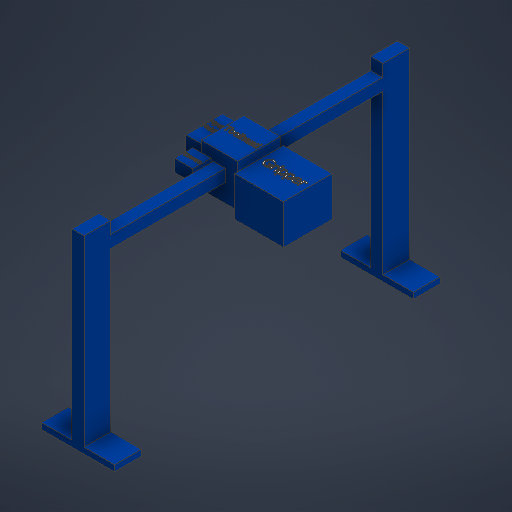
# Autodesk Inventor part: ToolheadMock
Saved by Autodesk Inventor 2025.1 (Build 291241000, 241)
## iProperties
Created: 2024-11-01
Part Number: ToolheadMock
Material: Generic
Document SubType Name: Modeling
Designer: jerem
Density: 1 g/cm^3
Appearance: Default
Author: jerem
Autodesk Inventor part; units mm, degrees
(part 1 of 2)
ref_plane "YZ Plane" through (0, 0, 0) normal (1, 0, 0) x (0, 1, 0)
ref_plane "XZ Plane" through (0, 0, 0) normal (0, 1, 0) x (-1, 0, 0)
sketch "Sketch1" plane through (0, 0, 0) normal (0, 1, 0) x (-1, 0, 0)
  line L0 (0, 0) -> (120, 0)
  line L1 (120, 0) -> (120, -44)
  line L2 (120, -44) -> (0, -44)
  line L3 (0, -44) -> (0, 0)
  line L4 (70, 0) -> (50, 0)
  line L5 (50, 0) -> (50, -44)
  line L6 (50, -44) -> (70, -44)
  line L7 (70, -44) -> (70, 0)
  point P0 (60, -44)
  dimension "d0" = 44
  dimension "d1" = 120
  dimension "d4" = 20
  dimension "d5" = 10
  constraints: 16 end point, 4 parallel, 2 horizontal, 2 perpendicular, 2 point on line, 1 midpoint
  measures "d0" distance of L0.end L1.end
  measures "d1" distance of L0.start L0.end
  measures "d4" distance between parallel lines of L5 L7
  measures "d5" distance from line of L5 point (60, -44)
extrude "Extrusion1" add sketch "Sketch1" along normal blind 10
extrude "Extrusion2" add sketch "Sketch1" along normal blind 300 from surface at 10 contours L0 L7 L2 L5
sketch "Sketch2" plane through (0, 0, -44) normal (0, 0, -1) x (-1, 0, 0)
  line L0 (50, 10) -> (50, 310) projected
  line L1 (70, 310) -> (70, 10) projected
  line L2 (50, 290) -> (70, 290)
  line L3 (70, 290) -> (70, 270)
  line L4 (70, 270) -> (50, 270)
  line L5 (50, 270) -> (50, 290)
  line L6 (70, 310) -> (50, 310) projected
  point P0 (0, 0)
  dimension "d8" = 20
  dimension "d9" = 20
  constraints: 8 end point, 2 parallel, 2 point on line, 1 horizontal, 1 perpendicular
  measures "d8" distance between parallel lines of L4 L2
  measures "d9" distance between parallel lines of L6 L2
extrude "Extrusion3" add sketch "Sketch2" along normal blind 445.8 contours L0 L2 L1 L4
ref_plane "Work Plane1" through (-50, 310, -266.9) normal (0, 0, -1) x (-1, 0, 0)
mirror "Mirror1" about plane through (-50, 310, -266.9) normal (0, 0, -1) of "Extrusion1", "Extrusion2"
sketch "Sketch3" plane through (-50, 310, -266.9) normal (0, 0, -1) x (-1, 0, 0)
  line L0 (40, 0) -> (-20, 0)
  line L1 (-20, 0) -> (-20, -70)
  line L2 (-20, -70) -> (40, -70)
  line L3 (40, -70) -> (40, 0)
  line L4 (20, 0) -> (20, -300) projected
  line L5 (0, -300) -> (0, 0) projected
  line L6 (20, -20) -> (0, -20) projected
  line L7 (0, -40) -> (20, -40) projected
  line L8 (40, -10) -> (70, -10)
  line L9 (70, -10) -> (70, -75)
  line L10 (70, -75) -> (40, -75)
  line L11 (40, -75) -> (40, -10)
  line L12 (-20, -15) -> (-100, -15)
  line L13 (-100, -15) -> (-100, -80)
  line L14 (-100, -80) -> (-20, -80)
  line L15 (-20, -80) -> (-20, -15)
  line L16 (23.5907, -17.4623) -> (53.5907, -17.4623)
  line L17 (53.5907, -17.4623) -> (53.5907, -37.4623)
  line L18 (53.5907, -37.4623) -> (23.5907, -37.4623)
  line L19 (23.5907, -37.4623) -> (23.5907, -17.4623)
  point P0 (-50, -310)
  point P1 (10, -20)
  point P2 (10, 0)
  point P3 (40, -70)
  point P4 (-20, -70)
  dimension "d12" = 20
  dimension "d13" = 20
  dimension "d14" = 20
  dimension "d15" = 30
  dimension "d16" = 10
  dimension "d17" = 15
  dimension "d18" = 10
  dimension "d19" = 80
  dimension "d20" = 30
  dimension "d41" = 5
  dimension "d42" = 30
  dimension "d43" = 20
  constraints: 32 end point, 8 parallel, 4 horizontal, 4 perpendicular, 2 midpoint, 2 point on line
  measures "d12" distance between parallel lines of L4 L3
  measures "d13" distance between parallel lines of L1 L5
  measures "d14" distance of point (10, -20) point (10, 0)
  measures "d15" distance between parallel lines of L2 L7
  measures "d16" distance from line of L0.start L8
  measures "d17" distance between parallel lines of L12 L0
  measures "d18" distance between parallel lines of L2 L14
  measures "d19" distance between parallel lines of L1 L13
  measures "d20" distance between parallel lines of L3 L9
  measures "d41" distance between parallel lines of L2 L10
  measures "d42" distance of L17.end L18.end
  measures "d43" distance of L16.end L17.end
extrude "Extrusion4" add sketch "Sketch3" along normal mid plane 70 contours L3 L16 L19 L18 L2 L4 L0 | L4 L6 L5 L0 | L5 L2 L1 L0 | L3 L18 L19 L16 | L4 L2 L5 L7
extrude "Extrusion5" add sketch "Sketch3" along normal mid plane 60 contours L8 L9 L10 L11 L3 L18 L17 L16 | L16 L17 L18 L3
extrude "Extrusion6" add sketch "Sketch3" along normal mid plane 80 contours L1 L15 L14 L13 L12
sketch "Sketch4" plane through (-30, 295, -306.9) normal (0, 1, 0) x (1, 0, 0)
  line L0 (6.4231, -29.5897) -> (62.2497, -29.5897) construction
  line L1 (62.2497, -29.5897) -> (62.2497, -34.515) construction
  line L2 (62.2497, -34.515) -> (6.4231, -34.515) construction
  line L3 (6.4231, -34.515) -> (6.4231, -29.5897) construction
  spline S0 degree 2 poles (14.227, -45.1488) (12.6346, -45.1488) (9.9969, -44.1764) (9.0487, -43.1918) knots 0 0 0 1 2 2 2
  spline S1 degree 2 poles (9.0487, -43.1918) (8.1006, -42.195) (7.0917, -39.2534) (7.0917, -37.345) knots 0 0 0 1 2 2 2
  spline S2 degree 2 poles (7.0917, -37.345) (7.0917, -35.5338) (8.1128, -32.6651) (9.0609, -31.644) knots 0 0 0 1 2 2 2
  spline S3 degree 2 poles (9.0609, -31.644) (9.9726, -30.6594) (12.6468, -29.5897) (14.2392, -29.5897) knots 0 0 0 1 2 2 2
  spline S4 degree 2 poles (14.2392, -29.5897) (15.005, -29.5897) (16.3907, -29.8085) (17.0228, -30.003) knots 0 0 0 1 2 2 2
  spline S5 degree 2 poles (17.0228, -30.003) (17.5333, -30.1488) (18.7732, -30.6837) (19.15, -30.8782) knots 0 0 0 1 2 2 2
  line L4 (19.15, -30.8782) -> (19.15, -33.285)
  line L5 (19.15, -33.285) -> (18.9799, -33.285)
  spline S6 degree 2 poles (18.9799, -33.285) (18.603, -32.9568) (17.8129, -32.3612) (17.0836, -32.0208) knots 0 0 0 1 2 2 2
  spline S7 degree 2 poles (17.0836, -32.0208) (16.4758, -31.7169) (14.9077, -31.3158) (14.0082, -31.3158) knots 0 0 0 1 2 2 2
  spline S8 degree 2 poles (14.0082, -31.3158) (11.8445, -31.3158) (9.1703, -34.5735) (9.1703, -37.2842) knots 0 0 0 1 2 2 2
  spline S9 degree 2 poles (9.1703, -37.2842) (9.1703, -38.7915) (9.8753, -41.0524) (10.5439, -41.8304) knots 0 0 0 1 2 2 2
  spline S10 degree 2 poles (10.5439, -41.8304) (11.1881, -42.6083) (13.0115, -43.4228) (14.1541, -43.4228) knots 0 0 0 1 2 2 2
  spline S11 degree 2 poles (14.1541, -43.4228) (14.9928, -43.4228) (16.6703, -43.1796) (17.2416, -42.9365) knots 0 0 0 1 2 2 2
  line L6 (17.2416, -42.9365) -> (17.2416, -39.0589)
  line L7 (17.2416, -39.0589) -> (13.7651, -39.0589)
  line L8 (13.7651, -39.0589) -> (13.7651, -37.3085)
  line L9 (13.7651, -37.3085) -> (19.2108, -37.3085)
  line L10 (19.2108, -37.3085) -> (19.2108, -43.8604)
  spline S12 degree 2 poles (19.2108, -43.8604) (18.834, -44.0305) (17.5455, -44.5532) (16.9985, -44.7112) knots 0 0 0 1 2 2 2
  spline S13 degree 2 poles (16.9985, -44.7112) (16.257, -44.93) (15.0658, -45.1488) (14.227, -45.1488) knots 0 0 0 1 2 2 2
  line L11 (27.5374, -35.631) -> (27.4402, -35.631)
  spline S14 degree 2 poles (27.4402, -35.631) (27.2214, -35.5702) (26.7473, -35.5459) (26.4191, -35.5459) knots 0 0 0 1 2 2 2
  spline S15 degree 2 poles (26.4191, -35.5459) (25.6533, -35.5459) (24.146, -36.2145) (23.4653, -36.8709) knots 0 0 0 1 2 2 2
  line L12 (23.4653, -36.8709) -> (23.4653, -44.8571)
  line L13 (23.4653, -44.8571) -> (21.569, -44.8571)
  line L14 (21.569, -44.8571) -> (21.569, -33.601)
  line L15 (21.569, -33.601) -> (23.4653, -33.601)
  line L16 (23.4653, -33.601) -> (23.4653, -35.2785)
  spline S16 degree 2 poles (23.4653, -35.2785) (24.4985, -34.3547) (26.0423, -33.601) (26.7716, -33.601) knots 0 0 0 1 2 2 2
  spline S17 degree 2 poles (26.7716, -33.601) (27.0633, -33.601) (27.3551, -33.6253) (27.5374, -33.6618) knots 0 0 0 1 2 2 2
  line L17 (27.5374, -33.6618) -> (27.5374, -35.631)
  line L18 (30.941, -44.8571) -> (29.0447, -44.8571)
  line L19 (29.0447, -44.8571) -> (29.0447, -33.601)
  line L20 (29.0447, -33.601) -> (30.941, -33.601)
  line L21 (30.941, -33.601) -> (30.941, -44.8571)
  line L22 (31.0747, -31.7291) -> (28.9231, -31.7291)
  line L23 (28.9231, -31.7291) -> (28.9231, -29.7599)
  line L24 (28.9231, -29.7599) -> (31.0747, -29.7599)
  line L25 (31.0747, -29.7599) -> (31.0747, -31.7291)
  spline S18 degree 2 poles (43.1573, -38.9252) (43.1573, -41.7453) (40.471, -45.0759) (38.4167, -45.0759) knots 0 0 0 1 2 2 2
  spline S19 degree 2 poles (38.4167, -45.0759) (37.5779, -45.0759) (36.2894, -44.6869) (35.6209, -44.2858) knots 0 0 0 1 2 2 2
  line L26 (35.6209, -44.2858) -> (35.6209, -49.0022)
  line L27 (35.6209, -49.0022) -> (33.7246, -49.0022)
  line L28 (33.7246, -49.0022) -> (33.7246, -33.601)
  line L29 (33.7246, -33.601) -> (35.6209, -33.601)
  line L30 (35.6209, -33.601) -> (35.6209, -34.7801)
  spline S20 degree 2 poles (35.6209, -34.7801) (36.3259, -34.1359) (38.052, -33.285) (39.0609, -33.285) knots 0 0 0 1 2 2 2
  spline S21 degree 2 poles (39.0609, -33.285) (40.9936, -33.285) (43.1573, -36.3482) (43.1573, -38.9252) knots 0 0 0 1 2 2 2
  spline S22 degree 2 poles (41.2003, -39.144) (41.2003, -37.2112) (39.9726, -35.084) (38.599, -35.084) knots 0 0 0 1 2 2 2
  spline S23 degree 2 poles (38.599, -35.084) (37.7967, -35.084) (36.2894, -35.8012) (35.6209, -36.3604) knots 0 0 0 1 2 2 2
  line L31 (35.6209, -36.3604) -> (35.6209, -42.7542)
  spline S24 degree 2 poles (35.6209, -42.7542) (36.3624, -43.1067) (37.4199, -43.3741) (38.1006, -43.3741) knots 0 0 0 1 2 2 2
  spline S25 degree 2 poles (38.1006, -43.3741) (39.5714, -43.3741) (41.2003, -41.2104) (41.2003, -39.144) knots 0 0 0 1 2 2 2
  spline S26 degree 2 poles (54.5593, -38.9252) (54.5593, -41.7453) (51.8729, -45.0759) (49.8186, -45.0759) knots 0 0 0 1 2 2 2
  spline S27 degree 2 poles (49.8186, -45.0759) (48.9799, -45.0759) (47.6914, -44.6869) (47.0228, -44.2858) knots 0 0 0 1 2 2 2
  line L32 (47.0228, -44.2858) -> (47.0228, -49.0022)
  line L33 (47.0228, -49.0022) -> (45.1265, -49.0022)
  line L34 (45.1265, -49.0022) -> (45.1265, -33.601)
  line L35 (45.1265, -33.601) -> (47.0228, -33.601)
  line L36 (47.0228, -33.601) -> (47.0228, -34.7801)
  spline S28 degree 2 poles (47.0228, -34.7801) (47.7278, -34.1359) (49.4539, -33.285) (50.4628, -33.285) knots 0 0 0 1 2 2 2
  spline S29 degree 2 poles (50.4628, -33.285) (52.3956, -33.285) (54.5593, -36.3482) (54.5593, -38.9252) knots 0 0 0 1 2 2 2
  spline S30 degree 2 poles (52.6022, -39.144) (52.6022, -37.2112) (51.3745, -35.084) (50.0009, -35.084) knots 0 0 0 1 2 2 2
  spline S31 degree 2 poles (50.0009, -35.084) (49.1987, -35.084) (47.6914, -35.8012) (47.0228, -36.3604) knots 0 0 0 1 2 2 2
  line L37 (47.0228, -36.3604) -> (47.0228, -42.7542)
  spline S32 degree 2 poles (47.0228, -42.7542) (47.7643, -43.1067) (48.8218, -43.3741) (49.5026, -43.3741) knots 0 0 0 1 2 2 2
  spline S33 degree 2 poles (49.5026, -43.3741) (50.9734, -43.3741) (52.6022, -41.2104) (52.6022, -39.144) knots 0 0 0 1 2 2 2
  spline S34 degree 2 poles (61.415, -45.1124) (58.7165, -45.1124) (55.7505, -42.0856) (55.7505, -39.2898) knots 0 0 0 1 2 2 2
  spline S35 degree 2 poles (55.7505, -39.2898) (55.7505, -36.5427) (58.6314, -33.285) (60.9531, -33.285) knots 0 0 0 1 2 2 2
  spline S36 degree 2 poles (60.9531, -33.285) (61.9985, -33.285) (63.6152, -33.8928) (64.2108, -34.537) knots 0 0 0 1 2 2 2
  spline S37 degree 2 poles (64.2108, -34.537) (64.8186, -35.1813) (65.4628, -37.0411) (65.4628, -38.3903) knots 0 0 0 1 2 2 2
  line L38 (65.4628, -38.3903) -> (65.4628, -39.4236)
  line L39 (65.4628, -39.4236) -> (57.6711, -39.4236)
  spline S38 degree 2 poles (57.6711, -39.4236) (57.6711, -41.3806) (59.6403, -43.4592) (61.3907, -43.4592) knots 0 0 0 1 2 2 2
  spline S39 degree 2 poles (61.3907, -43.4592) (62.0107, -43.4592) (63.2141, -43.1796) (63.7003, -42.9608) knots 0 0 0 1 2 2 2
  spline S40 degree 2 poles (63.7003, -42.9608) (64.2108, -42.7177) (64.9158, -42.2923) (65.1468, -42.0978) knots 0 0 0 1 2 2 2
  line L40 (65.1468, -42.0978) -> (65.2562, -42.0978)
  line L41 (65.2562, -42.0978) -> (65.2562, -44.1642)
  spline S41 degree 2 poles (65.2562, -44.1642) (64.928, -44.298) (63.9312, -44.6869) (63.5423, -44.7963) knots 0 0 0 1 2 2 2
  spline S42 degree 2 poles (63.5423, -44.7963) (62.9953, -44.9544) (62.0957, -45.1124) (61.415, -45.1124) knots 0 0 0 1 2 2 2
  spline S43 degree 2 poles (63.6152, -37.977) (63.5909, -37.2112) (63.2748, -36.0929) (62.971, -35.7161) knots 0 0 0 1 2 2 2
  spline S44 degree 2 poles (62.971, -35.7161) (62.6427, -35.2907) (61.6095, -34.8409) (60.8437, -34.8409) knots 0 0 0 1 2 2 2
  spline S45 degree 2 poles (60.8437, -34.8409) (60.0901, -34.8409) (59.0325, -35.2907) (58.5949, -35.7283) knots 0 0 0 1 2 2 2
  spline S46 degree 2 poles (58.5949, -35.7283) (58.1695, -36.178) (57.7319, -37.2599) (57.6711, -37.977) knots 0 0 0 1 2 2 2
  line L42 (57.6711, -37.977) -> (63.6152, -37.977)
  line L43 (73.3518, -35.631) -> (73.2546, -35.631)
  spline S47 degree 2 poles (73.2546, -35.631) (73.0358, -35.5702) (72.5617, -35.5459) (72.2335, -35.5459) knots 0 0 0 1 2 2 2
  spline S48 degree 2 poles (72.2335, -35.5459) (71.4677, -35.5459) (69.9604, -36.2145) (69.2797, -36.8709) knots 0 0 0 1 2 2 2
  line L44 (69.2797, -36.8709) -> (69.2797, -44.8571)
  line L45 (69.2797, -44.8571) -> (67.3834, -44.8571)
  line L46 (67.3834, -44.8571) -> (67.3834, -33.601)
  line L47 (67.3834, -33.601) -> (69.2797, -33.601)
  line L48 (69.2797, -33.601) -> (69.2797, -35.2785)
  spline S49 degree 2 poles (69.2797, -35.2785) (70.3129, -34.3547) (71.8567, -33.601) (72.586, -33.601) knots 0 0 0 1 2 2 2
  spline S50 degree 2 poles (72.586, -33.601) (72.8778, -33.601) (73.1695, -33.6253) (73.3518, -33.6618) knots 0 0 0 1 2 2 2
  line L49 (73.3518, -33.6618) -> (73.3518, -35.631)
  point P0 (30, -306.9)
  dimension "d0" = 44
  dimension "d1" = 120
  dimension "d4" = 20
  dimension "d5" = 10
  constraints: 2 other
sketch "Sketch5" plane through (-90, 310, -301.9) normal (0, 1, 0) x (1, 0, 0)
  line L0 (1.873, -26.5133) -> (57.6996, -26.5133) construction
  line L1 (57.6996, -26.5133) -> (57.6996, -37.1697) construction
  line L2 (57.6996, -37.1697) -> (1.873, -37.1697) construction
  line L3 (1.873, -37.1697) -> (1.873, -26.5133) construction
  line L4 (5.2198, -36.959) -> (5.2198, -28.1422)
  line L5 (5.2198, -28.1422) -> (1.8649, -28.1422)
  line L6 (1.8649, -28.1422) -> (1.8649, -26.959)
  line L7 (1.8649, -26.959) -> (9.9038, -26.959)
  line L8 (9.9038, -26.959) -> (9.9038, -28.1422)
  line L9 (9.9038, -28.1422) -> (6.5488, -28.1422)
  line L10 (6.5488, -28.1422) -> (6.5488, -36.959)
  line L11 (6.5488, -36.959) -> (5.2198, -36.959)
  spline S0 degree 2 poles (16.9864, -33.207) (16.9864, -35.1033) (15.1631, -37.1697) (13.6396, -37.1697) knots 0 0 0 1 2 2 2
  spline S1 degree 2 poles (13.6396, -37.1697) (12.0756, -37.1697) (10.2846, -35.0385) (10.2846, -33.207) knots 0 0 0 1 2 2 2
  spline S2 degree 2 poles (10.2846, -33.207) (10.2846, -31.3269) (12.1323, -29.2443) (13.6396, -29.2443) knots 0 0 0 1 2 2 2
  spline S3 degree 2 poles (13.6396, -29.2443) (15.1631, -29.2443) (16.9864, -31.3188) (16.9864, -33.207) knots 0 0 0 1 2 2 2
  spline S4 degree 2 poles (15.6817, -33.207) (15.6817, -31.7483) (14.6201, -30.3302) (13.6396, -30.3302) knots 0 0 0 1 2 2 2
  spline S5 degree 2 poles (13.6396, -30.3302) (12.659, -30.3302) (11.5893, -31.7483) (11.5893, -33.207) knots 0 0 0 1 2 2 2
  spline S6 degree 2 poles (11.5893, -33.207) (11.5893, -34.6252) (12.659, -36.0838) (13.6396, -36.0838) knots 0 0 0 1 2 2 2
  spline S7 degree 2 poles (13.6396, -36.0838) (14.612, -36.0838) (15.6817, -34.6495) (15.6817, -33.207) knots 0 0 0 1 2 2 2
  spline S8 degree 2 poles (24.45, -33.207) (24.45, -35.1033) (22.6266, -37.1697) (21.1031, -37.1697) knots 0 0 0 1 2 2 2
  spline S9 degree 2 poles (21.1031, -37.1697) (19.5391, -37.1697) (17.7482, -35.0385) (17.7482, -33.207) knots 0 0 0 1 2 2 2
  spline S10 degree 2 poles (17.7482, -33.207) (17.7482, -31.3269) (19.5958, -29.2443) (21.1031, -29.2443) knots 0 0 0 1 2 2 2
  spline S11 degree 2 poles (21.1031, -29.2443) (22.6266, -29.2443) (24.45, -31.3188) (24.45, -33.207) knots 0 0 0 1 2 2 2
  spline S12 degree 2 poles (23.1453, -33.207) (23.1453, -31.7483) (22.0837, -30.3302) (21.1031, -30.3302) knots 0 0 0 1 2 2 2
  spline S13 degree 2 poles (21.1031, -30.3302) (20.1226, -30.3302) (19.0529, -31.7483) (19.0529, -33.207) knots 0 0 0 1 2 2 2
  spline S14 degree 2 poles (19.0529, -33.207) (19.0529, -34.6252) (20.1226, -36.0838) (21.1031, -36.0838) knots 0 0 0 1 2 2 2
  spline S15 degree 2 poles (21.1031, -36.0838) (22.0756, -36.0838) (23.1453, -34.6495) (23.1453, -33.207) knots 0 0 0 1 2 2 2
  line L12 (27.0351, -36.959) -> (25.7709, -36.959)
  line L13 (25.7709, -36.959) -> (25.7709, -26.5133)
  line L14 (25.7709, -26.5133) -> (27.0351, -26.5133)
  line L15 (27.0351, -26.5133) -> (27.0351, -36.959)
  line L16 (34.7822, -36.959) -> (33.518, -36.959)
  line L17 (33.518, -36.959) -> (33.518, -32.6803)
  spline S16 degree 2 poles (33.518, -32.6803) (33.518, -32.1616) (33.4208, -31.2702) (33.2749, -31.0028) knots 0 0 0 1 2 2 2
  spline S17 degree 2 poles (33.2749, -31.0028) (33.121, -30.7192) (32.5699, -30.4436) (32.0999, -30.4436) knots 0 0 0 1 2 2 2
  spline S18 degree 2 poles (32.0999, -30.4436) (31.6299, -30.4436) (30.6331, -30.9461) (30.155, -31.3513) knots 0 0 0 1 2 2 2
  line L18 (30.155, -31.3513) -> (30.155, -36.959)
  line L19 (30.155, -36.959) -> (28.8908, -36.959)
  line L20 (28.8908, -36.959) -> (28.8908, -26.5133)
  line L21 (28.8908, -26.5133) -> (30.155, -26.5133)
  line L22 (30.155, -26.5133) -> (30.155, -30.2897)
  spline S19 degree 2 poles (30.155, -30.2897) (30.7223, -29.7791) (31.8163, -29.2443) (32.4321, -29.2443) knots 0 0 0 1 2 2 2
  spline S20 degree 2 poles (32.4321, -29.2443) (33.5342, -29.2443) (34.7822, -30.703) (34.7822, -32.0887) knots 0 0 0 1 2 2 2
  line L23 (34.7822, -32.0887) -> (34.7822, -36.959)
  spline S21 degree 2 poles (39.8146, -37.1292) (38.0156, -37.1292) (36.0383, -35.1114) (36.0383, -33.2475) knots 0 0 0 1 2 2 2
  spline S22 degree 2 poles (36.0383, -33.2475) (36.0383, -31.4161) (37.9589, -29.2443) (39.5067, -29.2443) knots 0 0 0 1 2 2 2
  spline S23 degree 2 poles (39.5067, -29.2443) (40.2036, -29.2443) (41.2814, -29.6495) (41.6785, -30.079) knots 0 0 0 1 2 2 2
  spline S24 degree 2 poles (41.6785, -30.079) (42.0837, -30.5085) (42.5132, -31.7483) (42.5132, -32.6479) knots 0 0 0 1 2 2 2
  line L24 (42.5132, -32.6479) -> (42.5132, -33.3367)
  line L25 (42.5132, -33.3367) -> (37.3187, -33.3367)
  spline S25 degree 2 poles (37.3187, -33.3367) (37.3187, -34.6414) (38.6315, -36.0271) (39.7984, -36.0271) knots 0 0 0 1 2 2 2
  spline S26 degree 2 poles (39.7984, -36.0271) (40.2117, -36.0271) (41.014, -35.8407) (41.3381, -35.6949) knots 0 0 0 1 2 2 2
  spline S27 degree 2 poles (41.3381, -35.6949) (41.6785, -35.5328) (42.1485, -35.2491) (42.3025, -35.1195) knots 0 0 0 1 2 2 2
  line L26 (42.3025, -35.1195) -> (42.3754, -35.1195)
  line L27 (42.3754, -35.1195) -> (42.3754, -36.4971)
  spline S28 degree 2 poles (42.3754, -36.4971) (42.1566, -36.5863) (41.4921, -36.8456) (41.2328, -36.9185) knots 0 0 0 1 2 2 2
  spline S29 degree 2 poles (41.2328, -36.9185) (40.8681, -37.0239) (40.2684, -37.1292) (39.8146, -37.1292) knots 0 0 0 1 2 2 2
  spline S30 degree 2 poles (41.2814, -32.3723) (41.2652, -31.8618) (41.0545, -31.1162) (40.8519, -30.865) knots 0 0 0 1 2 2 2
  spline S31 degree 2 poles (40.8519, -30.865) (40.6331, -30.5814) (39.9443, -30.2816) (39.4338, -30.2816) knots 0 0 0 1 2 2 2
  spline S32 degree 2 poles (39.4338, -30.2816) (38.9313, -30.2816) (38.2263, -30.5814) (37.9346, -30.8731) knots 0 0 0 1 2 2 2
  spline S33 degree 2 poles (37.9346, -30.8731) (37.6509, -31.173) (37.3592, -31.8942) (37.3187, -32.3723) knots 0 0 0 1 2 2 2
  line L28 (37.3187, -32.3723) -> (41.2814, -32.3723)
  spline S34 degree 2 poles (47.9751, -36.1649) (47.8211, -36.2783) (47.3025, -36.6835) (47.0594, -36.8051) knots 0 0 0 1 2 2 2
  spline S35 degree 2 poles (47.0594, -36.8051) (46.7271, -36.9833) (46.1031, -37.1697) (45.5359, -37.1697) knots 0 0 0 1 2 2 2
  spline S36 degree 2 poles (45.5359, -37.1697) (45.074, -37.1697) (44.2393, -36.8213) (43.9232, -36.5052) knots 0 0 0 1 2 2 2
  spline S37 degree 2 poles (43.9232, -36.5052) (43.6234, -36.1973) (43.2587, -35.2897) (43.2587, -34.7872) knots 0 0 0 1 2 2 2
  spline S38 degree 2 poles (43.2587, -34.7872) (43.2587, -34.0093) (43.9151, -32.9072) (44.6282, -32.5911) knots 0 0 0 1 2 2 2
  spline S39 degree 2 poles (44.6282, -32.5911) (45.2603, -32.2994) (46.9783, -32.0806) (47.9751, -32.0239) knots 0 0 0 1 2 2 2
  line L29 (47.9751, -32.0239) -> (47.9751, -31.7808)
  spline S40 degree 2 poles (47.9751, -31.7808) (47.9751, -31.3432) (47.7077, -30.8002) (47.4646, -30.6462) knots 0 0 0 1 2 2 2
  spline S41 degree 2 poles (47.4646, -30.6462) (47.2214, -30.4923) (46.5245, -30.395) (46.1517, -30.395) knots 0 0 0 1 2 2 2
  spline S42 degree 2 poles (46.1517, -30.395) (45.7141, -30.395) (44.531, -30.6543) (43.9394, -30.9056) knots 0 0 0 1 2 2 2
  line L30 (43.9394, -30.9056) -> (43.8665, -30.9056)
  line L31 (43.8665, -30.9056) -> (43.8665, -29.6171)
  spline S43 degree 2 poles (43.8665, -29.6171) (44.215, -29.5198) (45.5197, -29.2767) (46.1599, -29.2767) knots 0 0 0 1 2 2 2
  spline S44 degree 2 poles (46.1599, -29.2767) (46.9378, -29.2767) (47.9994, -29.5198) (48.4208, -29.8359) knots 0 0 0 1 2 2 2
  spline S45 degree 2 poles (48.4208, -29.8359) (48.8341, -30.1438) (49.2393, -31.1244) (49.2393, -31.8294) knots 0 0 0 1 2 2 2
  line L32 (49.2393, -31.8294) -> (49.2393, -36.959)
  line L33 (49.2393, -36.959) -> (47.9751, -36.959)
  line L34 (47.9751, -36.959) -> (47.9751, -36.1649)
  line L35 (47.9751, -35.1114) -> (47.9751, -33.0287)
  spline S46 degree 2 poles (47.9751, -33.0287) (47.5213, -33.0692) (46.1517, -33.207) (45.7223, -33.3367) knots 0 0 0 1 2 2 2
  spline S47 degree 2 poles (45.7223, -33.3367) (45.2198, -33.4906) (44.5634, -34.1308) (44.5634, -34.6981) knots 0 0 0 1 2 2 2
  spline S48 degree 2 poles (44.5634, -34.6981) (44.5634, -35.3464) (45.2928, -36.0028) (45.9897, -36.0028) knots 0 0 0 1 2 2 2
  spline S49 degree 2 poles (45.9897, -36.0028) (46.5812, -36.0028) (47.5537, -35.4923) (47.9751, -35.1114) knots 0 0 0 1 2 2 2
  line L36 (56.7838, -36.959) -> (55.5197, -36.959)
  line L37 (55.5197, -36.959) -> (55.5197, -36.1973)
  spline S50 degree 2 poles (55.5197, -36.1973) (55.2279, -36.4404) (54.7984, -36.7645) (54.5067, -36.9023) knots 0 0 0 1 2 2 2
  spline S51 degree 2 poles (54.5067, -36.9023) (54.2393, -37.032) (53.6639, -37.1697) (53.283, -37.1697) knots 0 0 0 1 2 2 2
  spline S52 degree 2 poles (53.283, -37.1697) (52.6671, -37.1697) (51.6299, -36.6592) (51.2652, -36.1649) knots 0 0 0 1 2 2 2
  spline S53 degree 2 poles (51.2652, -36.1649) (50.9005, -35.6705) (50.4953, -34.2119) (50.4953, -33.2637) knots 0 0 0 1 2 2 2
  spline S54 degree 2 poles (50.4953, -33.2637) (50.4953, -32.2751) (51.0059, -30.8326) (51.4516, -30.2897) knots 0 0 0 1 2 2 2
  spline S55 degree 2 poles (51.4516, -30.2897) (51.8649, -29.8034) (53.0237, -29.2443) (53.6639, -29.2443) knots 0 0 0 1 2 2 2
  spline S56 degree 2 poles (53.6639, -29.2443) (54.2231, -29.2443) (55.0577, -29.4955) (55.5197, -29.7548) knots 0 0 0 1 2 2 2
  line L38 (55.5197, -29.7548) -> (55.5197, -26.5133)
  line L39 (55.5197, -26.5133) -> (56.7838, -26.5133)
  line L40 (56.7838, -26.5133) -> (56.7838, -36.959)
  line L41 (55.5197, -35.1357) -> (55.5197, -30.8002)
  spline S57 degree 2 poles (55.5197, -30.8002) (55.0496, -30.5733) (54.3041, -30.4031) (53.8746, -30.4031) knots 0 0 0 1 2 2 2
  spline S58 degree 2 poles (53.8746, -30.4031) (52.9022, -30.4031) (51.8, -31.8618) (51.8, -33.2394) knots 0 0 0 1 2 2 2
  spline S59 degree 2 poles (51.8, -33.2394) (51.8, -34.5684) (52.6428, -35.9704) (53.5748, -35.9704) knots 0 0 0 1 2 2 2
  spline S60 degree 2 poles (53.5748, -35.9704) (54.0691, -35.9704) (55.074, -35.5166) (55.5197, -35.1357) knots 0 0 0 1 2 2 2
  point P0 (90, -301.9)
  dimension "d0" = 44
  dimension "d1" = 120
  dimension "d4" = 20
  dimension "d5" = 10
  constraints: 2 other
sketch "Sketch6" plane through (-120, 300, -296.9) normal (0, 1, 0) x (1, 0, 0)
  line L0 (0.0486, -16.372) -> (42.0583, -16.372) construction
  line L1 (42.0583, -16.372) -> (42.0583, -43.1123) construction
  line L2 (42.0583, -43.1123) -> (0.0486, -43.1123) construction
  line L3 (0.0486, -43.1123) -> (0.0486, -16.372) construction
  spline S0 degree 2 poles (5.1823, -18.5276) (5.1823, -18.9814) (4.859, -19.7983) (4.5697, -20.0819) knots 0 0 0 1 2 2 2
  spline S1 degree 2 poles (4.5697, -20.0819) (4.2066, -20.4393) (3.2253, -20.808) (2.4765, -20.808) knots 0 0 0 1 2 2 2
  line L4 (2.4765, -20.808) -> (1.688, -20.808)
  line L5 (1.688, -20.808) -> (1.688, -23.4174)
  line L6 (1.688, -23.4174) -> (0.7577, -23.4174)
  line L7 (0.7577, -23.4174) -> (0.7577, -16.4174)
  line L8 (0.7577, -16.4174) -> (2.5162, -16.4174)
  spline S2 degree 2 poles (2.5162, -16.4174) (3.1402, -16.4174) (4.0138, -16.6216) (4.3485, -16.8542) knots 0 0 0 1 2 2 2
  spline S3 degree 2 poles (4.3485, -16.8542) (4.7399, -17.1208) (5.1823, -17.9434) (5.1823, -18.5276) knots 0 0 0 1 2 2 2
  spline S4 degree 2 poles (4.2123, -18.556) (4.2123, -18.1929) (3.9627, -17.6597) (3.7074, -17.4895) knots 0 0 0 1 2 2 2
  spline S5 degree 2 poles (3.7074, -17.4895) (3.4862, -17.3421) (2.8963, -17.2229) (2.4595, -17.2229) knots 0 0 0 1 2 2 2
  line L9 (2.4595, -17.2229) -> (1.688, -17.2229)
  line L10 (1.688, -17.2229) -> (1.688, -20.0139)
  line L11 (1.688, -20.0139) -> (2.3233, -20.0139)
  spline S6 degree 2 poles (2.3233, -20.0139) (2.8906, -20.0139) (3.5883, -19.8323) (3.8152, -19.5941) knots 0 0 0 1 2 2 2
  spline S7 degree 2 poles (3.8152, -19.5941) (4.0251, -19.3842) (4.2123, -18.8907) (4.2123, -18.556) knots 0 0 0 1 2 2 2
  line L12 (6.9011, -23.4174) -> (6.0162, -23.4174)
  line L13 (6.0162, -23.4174) -> (6.0162, -18.1646)
  line L14 (6.0162, -18.1646) -> (6.9011, -18.1646)
  line L15 (6.9011, -18.1646) -> (6.9011, -23.4174)
  line L16 (6.9635, -17.291) -> (5.9595, -17.291)
  line L17 (5.9595, -17.291) -> (5.9595, -16.372)
  line L18 (5.9595, -16.372) -> (6.9635, -16.372)
  line L19 (6.9635, -16.372) -> (6.9635, -17.291)
  spline S8 degree 2 poles (12.6021, -20.6492) (12.6021, -21.9652) (11.3485, -23.5195) (10.3898, -23.5195) knots 0 0 0 1 2 2 2
  spline S9 degree 2 poles (10.3898, -23.5195) (9.9984, -23.5195) (9.3971, -23.338) (9.0851, -23.1508) knots 0 0 0 1 2 2 2
  line L20 (9.0851, -23.1508) -> (9.0851, -25.3518)
  line L21 (9.0851, -25.3518) -> (8.2002, -25.3518)
  line L22 (8.2002, -25.3518) -> (8.2002, -18.1646)
  line L23 (8.2002, -18.1646) -> (9.0851, -18.1646)
  line L24 (9.0851, -18.1646) -> (9.0851, -18.7148)
  spline S10 degree 2 poles (9.0851, -18.7148) (9.4141, -18.4142) (10.2196, -18.0171) (10.6904, -18.0171) knots 0 0 0 1 2 2 2
  spline S11 degree 2 poles (10.6904, -18.0171) (11.5924, -18.0171) (12.6021, -19.4466) (12.6021, -20.6492) knots 0 0 0 1 2 2 2
  spline S12 degree 2 poles (11.6888, -20.7513) (11.6888, -19.8493) (11.1159, -18.8566) (10.4749, -18.8566) knots 0 0 0 1 2 2 2
  spline S13 degree 2 poles (10.4749, -18.8566) (10.1005, -18.8566) (9.3971, -19.1913) (9.0851, -19.4523) knots 0 0 0 1 2 2 2
  line L25 (9.0851, -19.4523) -> (9.0851, -22.4361)
  spline S14 degree 2 poles (9.0851, -22.4361) (9.4311, -22.6006) (9.9246, -22.7254) (10.2423, -22.7254) knots 0 0 0 1 2 2 2
  spline S15 degree 2 poles (10.2423, -22.7254) (10.9287, -22.7254) (11.6888, -21.7156) (11.6888, -20.7513) knots 0 0 0 1 2 2 2
  spline S16 degree 2 poles (15.8015, -23.5365) (14.5421, -23.5365) (13.158, -22.1241) (13.158, -20.8194) knots 0 0 0 1 2 2 2
  spline S17 degree 2 poles (13.158, -20.8194) (13.158, -19.5374) (14.5024, -18.0171) (15.5859, -18.0171) knots 0 0 0 1 2 2 2
  spline S18 degree 2 poles (15.5859, -18.0171) (16.0737, -18.0171) (16.8282, -18.3007) (17.1062, -18.6014) knots 0 0 0 1 2 2 2
  spline S19 degree 2 poles (17.1062, -18.6014) (17.3898, -18.902) (17.6904, -19.7699) (17.6904, -20.3996) knots 0 0 0 1 2 2 2
  line L26 (17.6904, -20.3996) -> (17.6904, -20.8818)
  line L27 (17.6904, -20.8818) -> (14.0543, -20.8818)
  spline S20 degree 2 poles (14.0543, -20.8818) (14.0543, -21.7951) (14.9732, -22.7651) (15.7901, -22.7651) knots 0 0 0 1 2 2 2
  spline S21 degree 2 poles (15.7901, -22.7651) (16.0794, -22.7651) (16.641, -22.6346) (16.8679, -22.5325) knots 0 0 0 1 2 2 2
  spline S22 degree 2 poles (16.8679, -22.5325) (17.1062, -22.419) (17.4352, -22.2205) (17.5429, -22.1297) knots 0 0 0 1 2 2 2
  line L28 (17.5429, -22.1297) -> (17.594, -22.1297)
  line L29 (17.594, -22.1297) -> (17.594, -23.0941)
  spline S23 degree 2 poles (17.594, -23.0941) (17.4408, -23.1565) (16.9757, -23.338) (16.7942, -23.3891) knots 0 0 0 1 2 2 2
  spline S24 degree 2 poles (16.7942, -23.3891) (16.5389, -23.4628) (16.1191, -23.5365) (15.8015, -23.5365) knots 0 0 0 1 2 2 2
  spline S25 degree 2 poles (16.8282, -20.2067) (16.8168, -19.8493) (16.6694, -19.3275) (16.5275, -19.1516) knots 0 0 0 1 2 2 2
  spline S26 degree 2 poles (16.5275, -19.1516) (16.3744, -18.9531) (15.8922, -18.7432) (15.5348, -18.7432) knots 0 0 0 1 2 2 2
  spline S27 degree 2 poles (15.5348, -18.7432) (15.1831, -18.7432) (14.6896, -18.9531) (14.4854, -19.1573) knots 0 0 0 1 2 2 2
  spline S28 degree 2 poles (14.4854, -19.1573) (14.2869, -19.3672) (14.0826, -19.872) (14.0543, -20.2067) knots 0 0 0 1 2 2 2
  line L30 (14.0543, -20.2067) -> (16.8282, -20.2067)
  spline S29 degree 2 poles (20.175, -23.5195) (19.4546, -23.5195) (18.6434, -22.697) (18.6434, -21.8064) knots 0 0 0 1 2 2 2
  line L31 (18.6434, -21.8064) -> (18.6434, -18.8964)
  line L32 (18.6434, -18.8964) -> (18.0478, -18.8964)
  line L33 (18.0478, -18.8964) -> (18.0478, -18.1646)
  line L34 (18.0478, -18.1646) -> (18.6434, -18.1646)
  line L35 (18.6434, -18.1646) -> (18.6434, -16.6557)
  line L36 (18.6434, -16.6557) -> (19.5284, -16.6557)
  line L37 (19.5284, -16.6557) -> (19.5284, -18.1646)
  line L38 (19.5284, -18.1646) -> (21.1564, -18.1646)
  line L39 (21.1564, -18.1646) -> (21.1564, -18.8964)
  line L40 (21.1564, -18.8964) -> (19.5284, -18.8964)
  line L41 (19.5284, -18.8964) -> (19.5284, -21.398)
  spline S30 degree 2 poles (19.5284, -21.398) (19.5284, -21.7951) (19.5567, -22.2318) (19.6532, -22.419) knots 0 0 0 1 2 2 2
  spline S31 degree 2 poles (19.6532, -22.419) (19.7326, -22.5835) (20.0899, -22.7481) (20.3963, -22.7481) knots 0 0 0 1 2 2 2
  spline S32 degree 2 poles (20.3963, -22.7481) (20.6118, -22.7481) (21.0146, -22.6176) (21.1053, -22.5779) knots 0 0 0 1 2 2 2
  line L42 (21.1053, -22.5779) -> (21.1564, -22.5779)
  line L43 (21.1564, -22.5779) -> (21.1564, -23.372)
  spline S33 degree 2 poles (21.1564, -23.372) (20.9068, -23.4401) (20.3963, -23.5195) (20.175, -23.5195) knots 0 0 0 1 2 2 2
  spline S34 degree 2 poles (23.3971, -23.5195) (22.6767, -23.5195) (21.8655, -22.697) (21.8655, -21.8064) knots 0 0 0 1 2 2 2
  line L44 (21.8655, -21.8064) -> (21.8655, -18.8964)
  line L45 (21.8655, -18.8964) -> (21.2698, -18.8964)
  line L46 (21.2698, -18.8964) -> (21.2698, -18.1646)
  line L47 (21.2698, -18.1646) -> (21.8655, -18.1646)
  line L48 (21.8655, -18.1646) -> (21.8655, -16.6557)
  line L49 (21.8655, -16.6557) -> (22.7504, -16.6557)
  line L50 (22.7504, -16.6557) -> (22.7504, -18.1646)
  line L51 (22.7504, -18.1646) -> (24.3784, -18.1646)
  line L52 (24.3784, -18.1646) -> (24.3784, -18.8964)
  line L53 (24.3784, -18.8964) -> (22.7504, -18.8964)
  line L54 (22.7504, -18.8964) -> (22.7504, -21.398)
  spline S35 degree 2 poles (22.7504, -21.398) (22.7504, -21.7951) (22.7788, -22.2318) (22.8752, -22.419) knots 0 0 0 1 2 2 2
  spline S36 degree 2 poles (22.8752, -22.419) (22.9546, -22.5835) (23.312, -22.7481) (23.6183, -22.7481) knots 0 0 0 1 2 2 2
  spline S37 degree 2 poles (23.6183, -22.7481) (23.8339, -22.7481) (24.2366, -22.6176) (24.3274, -22.5779) knots 0 0 0 1 2 2 2
  line L55 (24.3274, -22.5779) -> (24.3784, -22.5779)
  line L56 (24.3784, -22.5779) -> (24.3784, -23.372)
  spline S38 degree 2 poles (24.3784, -23.372) (24.1288, -23.4401) (23.6183, -23.5195) (23.3971, -23.5195) knots 0 0 0 1 2 2 2
  spline S39 degree 2 poles (27.3112, -23.5365) (26.0519, -23.5365) (24.6677, -22.1241) (24.6677, -20.8194) knots 0 0 0 1 2 2 2
  spline S40 degree 2 poles (24.6677, -20.8194) (24.6677, -19.5374) (26.0121, -18.0171) (27.0956, -18.0171) knots 0 0 0 1 2 2 2
  spline S41 degree 2 poles (27.0956, -18.0171) (27.5835, -18.0171) (28.3379, -18.3007) (28.6159, -18.6014) knots 0 0 0 1 2 2 2
  spline S42 degree 2 poles (28.6159, -18.6014) (28.8995, -18.902) (29.2002, -19.7699) (29.2002, -20.3996) knots 0 0 0 1 2 2 2
  line L57 (29.2002, -20.3996) -> (29.2002, -20.8818)
  line L58 (29.2002, -20.8818) -> (25.564, -20.8818)
  spline S43 degree 2 poles (25.564, -20.8818) (25.564, -21.7951) (26.483, -22.7651) (27.2998, -22.7651) knots 0 0 0 1 2 2 2
  spline S44 degree 2 poles (27.2998, -22.7651) (27.5891, -22.7651) (28.1507, -22.6346) (28.3776, -22.5325) knots 0 0 0 1 2 2 2
  spline S45 degree 2 poles (28.3776, -22.5325) (28.6159, -22.419) (28.9449, -22.2205) (29.0527, -22.1297) knots 0 0 0 1 2 2 2
  line L59 (29.0527, -22.1297) -> (29.1037, -22.1297)
  line L60 (29.1037, -22.1297) -> (29.1037, -23.0941)
  spline S46 degree 2 poles (29.1037, -23.0941) (28.9506, -23.1565) (28.4854, -23.338) (28.3039, -23.3891) knots 0 0 0 1 2 2 2
  spline S47 degree 2 poles (28.3039, -23.3891) (28.0486, -23.4628) (27.6288, -23.5365) (27.3112, -23.5365) knots 0 0 0 1 2 2 2
  spline S48 degree 2 poles (28.3379, -20.2067) (28.3266, -19.8493) (28.1791, -19.3275) (28.0373, -19.1516) knots 0 0 0 1 2 2 2
  spline S49 degree 2 poles (28.0373, -19.1516) (27.8841, -18.9531) (27.4019, -18.7432) (27.0446, -18.7432) knots 0 0 0 1 2 2 2
  spline S50 degree 2 poles (27.0446, -18.7432) (26.6929, -18.7432) (26.1993, -18.9531) (25.9951, -19.1573) knots 0 0 0 1 2 2 2
  spline S51 degree 2 poles (25.9951, -19.1573) (25.7966, -19.3672) (25.5924, -19.872) (25.564, -20.2067) knots 0 0 0 1 2 2 2
  line L61 (25.564, -20.2067) -> (28.3379, -20.2067)
  line L62 (5.8403, -34.9427) -> (4.91, -34.9427)
  line L63 (4.91, -34.9427) -> (4.91, -31.5165)
  line L64 (4.91, -31.5165) -> (1.688, -31.5165)
  line L65 (1.688, -31.5165) -> (1.688, -34.9427)
  line L66 (1.688, -34.9427) -> (0.7577, -34.9427)
  line L67 (0.7577, -34.9427) -> (0.7577, -27.9427)
  line L68 (0.7577, -27.9427) -> (1.688, -27.9427)
  line L69 (1.688, -27.9427) -> (1.688, -30.6883)
  line L70 (1.688, -30.6883) -> (4.91, -30.6883)
  line L71 (4.91, -30.6883) -> (4.91, -27.9427)
  line L72 (4.91, -27.9427) -> (5.8403, -27.9427)
  line L73 (5.8403, -27.9427) -> (5.8403, -34.9427)
  spline S52 degree 2 poles (11.5073, -32.3163) (11.5073, -33.6437) (10.2309, -35.0902) (9.1645, -35.0902) knots 0 0 0 1 2 2 2
  spline S53 degree 2 poles (9.1645, -35.0902) (8.0697, -35.0902) (6.816, -33.5983) (6.816, -32.3163) knots 0 0 0 1 2 2 2
  spline S54 degree 2 poles (6.816, -32.3163) (6.816, -31.0003) (8.1094, -29.5424) (9.1645, -29.5424) knots 0 0 0 1 2 2 2
  spline S55 degree 2 poles (9.1645, -29.5424) (10.2309, -29.5424) (11.5073, -30.9946) (11.5073, -32.3163) knots 0 0 0 1 2 2 2
  spline S56 degree 2 poles (10.594, -32.3163) (10.594, -31.2952) (9.8509, -30.3025) (9.1645, -30.3025) knots 0 0 0 1 2 2 2
  spline S57 degree 2 poles (9.1645, -30.3025) (8.4781, -30.3025) (7.7293, -31.2952) (7.7293, -32.3163) knots 0 0 0 1 2 2 2
  spline S58 degree 2 poles (7.7293, -32.3163) (7.7293, -33.309) (8.4781, -34.3301) (9.1645, -34.3301) knots 0 0 0 1 2 2 2
  spline S59 degree 2 poles (9.1645, -34.3301) (9.8452, -34.3301) (10.594, -33.326) (10.594, -32.3163) knots 0 0 0 1 2 2 2
  line L74 (13.3168, -34.9427) -> (12.4319, -34.9427)
  line L75 (12.4319, -34.9427) -> (12.4319, -27.6307)
  line L76 (12.4319, -27.6307) -> (13.3168, -27.6307)
  line L77 (13.3168, -27.6307) -> (13.3168, -34.9427)
  line L78 (18.6548, -34.9427) -> (17.7698, -34.9427)
  line L79 (17.7698, -34.9427) -> (17.7698, -34.4095)
  spline S60 degree 2 poles (17.7698, -34.4095) (17.5656, -34.5797) (17.265, -34.8066) (17.0608, -34.903) knots 0 0 0 1 2 2 2
  spline S61 degree 2 poles (17.0608, -34.903) (16.8736, -34.9938) (16.4708, -35.0902) (16.2042, -35.0902) knots 0 0 0 1 2 2 2
  spline S62 degree 2 poles (16.2042, -35.0902) (15.7731, -35.0902) (15.047, -34.7328) (14.7917, -34.3868) knots 0 0 0 1 2 2 2
  spline S63 degree 2 poles (14.7917, -34.3868) (14.5365, -34.0408) (14.2528, -33.0197) (14.2528, -32.356) knots 0 0 0 1 2 2 2
  spline S64 degree 2 poles (14.2528, -32.356) (14.2528, -31.664) (14.6102, -30.6542) (14.9222, -30.2742) knots 0 0 0 1 2 2 2
  spline S65 degree 2 poles (14.9222, -30.2742) (15.2115, -29.9338) (16.0227, -29.5424) (16.4708, -29.5424) knots 0 0 0 1 2 2 2
  spline S66 degree 2 poles (16.4708, -29.5424) (16.8622, -29.5424) (17.4465, -29.7183) (17.7698, -29.8998) knots 0 0 0 1 2 2 2
  line L80 (17.7698, -29.8998) -> (17.7698, -27.6307)
  line L81 (17.7698, -27.6307) -> (18.6548, -27.6307)
  line L82 (18.6548, -27.6307) -> (18.6548, -34.9427)
  line L83 (17.7698, -33.6664) -> (17.7698, -30.6316)
  spline S67 degree 2 poles (17.7698, -30.6316) (17.4408, -30.4727) (16.919, -30.3536) (16.6183, -30.3536) knots 0 0 0 1 2 2 2
  spline S68 degree 2 poles (16.6183, -30.3536) (15.9376, -30.3536) (15.1661, -31.3747) (15.1661, -32.339) knots 0 0 0 1 2 2 2
  spline S69 degree 2 poles (15.1661, -32.339) (15.1661, -33.2693) (15.7561, -34.2507) (16.4084, -34.2507) knots 0 0 0 1 2 2 2
  spline S70 degree 2 poles (16.4084, -34.2507) (16.7544, -34.2507) (17.4579, -33.933) (17.7698, -33.6664) knots 0 0 0 1 2 2 2
  spline S71 degree 2 poles (22.2172, -35.0619) (20.9579, -35.0619) (19.5737, -33.6494) (19.5737, -32.3447) knots 0 0 0 1 2 2 2
  spline S72 degree 2 poles (19.5737, -32.3447) (19.5737, -31.0627) (20.9181, -29.5424) (22.0016, -29.5424) knots 0 0 0 1 2 2 2
  spline S73 degree 2 poles (22.0016, -29.5424) (22.4895, -29.5424) (23.2439, -29.826) (23.5219, -30.1267) knots 0 0 0 1 2 2 2
  spline S74 degree 2 poles (23.5219, -30.1267) (23.8055, -30.4273) (24.1062, -31.2952) (24.1062, -31.9249) knots 0 0 0 1 2 2 2
  line L84 (24.1062, -31.9249) -> (24.1062, -32.4071)
  line L85 (24.1062, -32.4071) -> (20.47, -32.4071)
  spline S75 degree 2 poles (20.47, -32.4071) (20.47, -33.3204) (21.389, -34.2904) (22.2058, -34.2904) knots 0 0 0 1 2 2 2
  spline S76 degree 2 poles (22.2058, -34.2904) (22.4951, -34.2904) (23.0567, -34.1599) (23.2836, -34.0578) knots 0 0 0 1 2 2 2
  spline S77 degree 2 poles (23.2836, -34.0578) (23.5219, -33.9444) (23.8509, -33.7458) (23.9587, -33.6551) knots 0 0 0 1 2 2 2
  line L86 (23.9587, -33.6551) -> (24.0097, -33.6551)
  line L87 (24.0097, -33.6551) -> (24.0097, -34.6194)
  spline S78 degree 2 poles (24.0097, -34.6194) (23.8566, -34.6818) (23.3914, -34.8633) (23.2099, -34.9144) knots 0 0 0 1 2 2 2
  spline S79 degree 2 poles (23.2099, -34.9144) (22.9546, -34.9881) (22.5348, -35.0619) (22.2172, -35.0619) knots 0 0 0 1 2 2 2
  spline S80 degree 2 poles (23.2439, -31.732) (23.2326, -31.3747) (23.0851, -30.8528) (22.9433, -30.6769) knots 0 0 0 1 2 2 2
  spline S81 degree 2 poles (22.9433, -30.6769) (22.7901, -30.4784) (22.3079, -30.2685) (21.9506, -30.2685) knots 0 0 0 1 2 2 2
  spline S82 degree 2 poles (21.9506, -30.2685) (21.5989, -30.2685) (21.1053, -30.4784) (20.9011, -30.6826) knots 0 0 0 1 2 2 2
  spline S83 degree 2 poles (20.9011, -30.6826) (20.7026, -30.8925) (20.4984, -31.3974) (20.47, -31.732) knots 0 0 0 1 2 2 2
  line L88 (20.47, -31.732) -> (23.2439, -31.732)
  line L89 (27.7877, -30.6372) -> (27.7423, -30.6372)
  spline S84 degree 2 poles (27.7423, -30.6372) (27.6402, -30.6089) (27.419, -30.5975) (27.2658, -30.5975) knots 0 0 0 1 2 2 2
  spline S85 degree 2 poles (27.2658, -30.5975) (26.9084, -30.5975) (26.205, -30.9095) (25.8873, -31.2158) knots 0 0 0 1 2 2 2
  line L90 (25.8873, -31.2158) -> (25.8873, -34.9427)
  line L91 (25.8873, -34.9427) -> (25.0024, -34.9427)
  line L92 (25.0024, -34.9427) -> (25.0024, -29.6899)
  line L93 (25.0024, -29.6899) -> (25.8873, -29.6899)
  line L94 (25.8873, -29.6899) -> (25.8873, -30.4727)
  spline S86 degree 2 poles (25.8873, -30.4727) (26.3695, -30.0416) (27.0899, -29.6899) (27.4303, -29.6899) knots 0 0 0 1 2 2 2
  spline S87 degree 2 poles (27.4303, -29.6899) (27.5664, -29.6899) (27.7026, -29.7012) (27.7877, -29.7183) knots 0 0 0 1 2 2 2
  line L95 (27.7877, -29.7183) -> (27.7877, -30.6372)
  point P0 (120, -296.9)
  dimension "d0" = 44
  dimension "d1" = 120
  dimension "d4" = 20
  dimension "d5" = 10
  constraints: 2 other
extrude "Extrusion7" add sketch "Sketch6" along normal mid plane 2
extrude "Extrusion8" add sketch "Sketch5" along normal mid plane 2
extrude "Extrusion9" add sketch "Sketch4" along normal mid plane 2
extrude "Extrusion10" add sketch "Sketch3" against normal blind 30 from surface at -35 contours L16 L17 L18 L3 | L3 L18 L19 L16